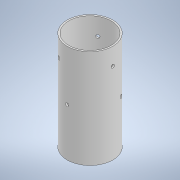
# Autodesk Inventor part: avbay
Saved by Autodesk Inventor 2020 (Build 240168000, 168)
## iProperties
Created: 2020-10-12
Part Number: avbay
Material: Generic
Document SubType Name: Modeling
Designer: mulve
Density: 1 g/cm^3
Appearance: Default
Author: mulve
Autodesk Inventor part; units mm, degrees
ref_plane "YZ Plane" through (0, 0, 0) normal (1, 0, 0) x (0, 1, 0)
sketch "Sketch1" plane through (0, 0, 0) normal (0, 1, 0) x (-1, 0, 0)
  circle A0 centre (0, 0) radius 27.31
  circle A1 centre (0, 0) radius 25.445
  dimension "d0" = 54.62
  dimension "d1" = 50.89
  constraints: 2 centre point, 2 coincident
  measures "d0" diameter of A0
  measures "d1" diameter of A1
extrude "Extrusion1" add sketch "Sketch1" along normal blind 115.81
sketch "Sketch2" plane through (0, 0, 0) normal (0, -1, 0) x (1, 0, 0)
  circle A0 centre (0, 0) radius 27.31
  constraints: 1 centre point, 1 coincident
extrude "Extrusion2" add sketch "Sketch2" along normal blind 2.18
sketch "Sketch3" plane through (0, -2.18, 0) normal (0, -1, 0) x (1, 0, 0)
  circle A0 centre (0, 0) radius 2.75
  dimension "d6" = 5.5
  constraints: 1 centre point, 1 coincident
  measures "d6" diameter of A0
extrude "Extrusion3" cut sketch "Sketch3" against normal up to surface (2.18 mm away)
sketch "Sketch4" plane through (0, 0, 0) normal (0, 1, 0) x (1, 0, 0)
  circle A0 centre (0, 0) radius 2.75 projected
  circle A1 centre (0, 0) radius 25.445
  circle A2 centre (0, 0) radius 2.75
  constraints: 2 centre point, 2 coincident, 1 concentric
extrude "Extrusion4" add sketch "Sketch4" along normal blind 2.56
ref_plane "Work Plane1" through (0, 95.06, 0) normal (0, 1, 0) x (1, 0, 0)
sketch "Sketch6" plane through (0, 95.06, 0) normal (0, 1, 0) x (1, 0, 0)
  circle A0 centre (0, 0) radius 27.31 projected
  point P0 (27.31, 0)
  point P1 (-13.655, 23.6512)
  point P2 (-13.655, -23.6512)
  dimension "d18" = 360
  constraints: 1 horizontal alignment, 5 other
hole "Hole1" at (-13.655, 95.06, -23.6512) direction (0.5, 0, 0.866) diameter 4.1 depth 2
hole "Hole2" at (-13.655, 95.06, 23.6512) direction (0.5, 0, -0.866) diameter 4.1 depth 2
hole "Hole3" at (27.31, 95.06, 0) direction (-1, 0, 0) diameter 4.1 depth 2
ref_plane "Work Plane2" through (0, 55.16, 0) normal (0, 1, 0) x (1, 0, 0)
sketch "Sketch7" plane through (0, 55.16, 0) normal (0, 1, 0) x (1, 0, 0)
  circle A0 centre (0, 0) radius 27.31 projected
  point P0 (0, -27.31)
  point P1 (23.6512, 13.655)
  point P2 (-23.6512, 13.655)
  dimension "d50" = 360
  constraints: 1 vertical alignment, 5 other
hole "Hole4" at (23.6512, 55.16, -13.655) direction (-0.866, 0, 0.5) diameter 4.1 depth 2
hole "Hole5" at (0, 55.16, 27.31) direction (0, 0, -1) diameter 4.1 depth 2
hole "Hole6" at (-23.6512, 55.16, -13.655) direction (0.866, 0, 0.5) diameter 4.1 depth 2
sketch "Sketch8" plane through (0, 2.56, 0) normal (0, 1, 0) x (1, 0, 0)
  circle A0 centre (0, 0) radius 2.75
  circle A1 centre (0, 0) radius 2.75 projected
  line L0 (-4.8047, 0) -> (-2.4023, 4.161)
  line L1 (-2.4023, 4.161) -> (2.4023, 4.161)
  line L2 (2.4023, 4.161) -> (4.8047, 0)
  line L3 (4.8047, 0) -> (2.4023, -4.161)
  line L4 (2.4023, -4.161) -> (-2.4023, -4.161)
  line L5 (-2.4023, -4.161) -> (-4.8047, 0)
  constraints: 12 end point, 2 coincident, 1 centre point, 1 concentric, 13 other
extrude "Extrusion5" add sketch "Sketch8" along normal blind 22.06 contours A0
extrude "Extrusion6" add sketch "Sketch8" along normal blind 3.175
ref_plane "Work Plane3" through (-2.4023, 2.56, -0.919) normal (0, 0, 1) x (1, 0, 0)
body "Solid1"
